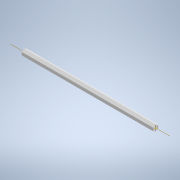
# Autodesk Inventor part: HexShaft
Saved by Autodesk Inventor 2020.2 (Build 242310000, 310)
## iProperties
Created: 2020-02-11
Part Number: HexShaft
Material: Generic
Document SubType Name: Modeling
Designer: AOFUser
Density: 1 g/cm^3
Appearance: Default
Author: AOFUser
Autodesk Inventor part; units mm, degrees
ref_plane "YZ Plane" through (0, 0, 0) normal (1, 0, 0) x (0, 1, 0)
ref_plane "XZ Plane" through (0, 0, 0) normal (0, 1, 0) x (-1, 0, 0)
ref_plane "XY Plane" through (0, 0, 0) normal (0, 0, 1) x (1, 0, 0)
sketch "Sketch1" plane through (0, 0, 0) normal (1, 0, 0) x (0, 1, 0)
  line L0 (-1.5584, 2.6992) -> (-3.1168, 0)
  line L1 (1.5584, 2.6992) -> (-1.5584, 2.6992)
  line L2 (3.1168, 0) -> (1.5584, 2.6992)
  line L3 (1.5584, -2.6992) -> (3.1168, 0)
  line L4 (-1.5584, -2.6992) -> (1.5584, -2.6992)
  line L5 (-3.1168, 0) -> (-1.5584, -2.6992)
  point P0 (0, 0)
  point P1 (0, 0)
  point P2 (0, 0)
  constraints: 12 end point, 1 coincident
extrude "Extrusion1" add sketch "Sketch1" along normal blind 134.9375
sketch "Sketch2" plane through (0, 0, 0) normal (-1, 0, 0) x (0, 0, 1)
  point P0 (0, 0)
  point P1 (0, 0)
  constraints: 1 coincident
sketch "Sketch3" plane through (134.9375, 0, 0) normal (1, 0, 0) x (0, 0, -1)
  point P0 (0, 0)
  point P1 (0, 0)
  constraints: 1 coincident
body "Solid1"
